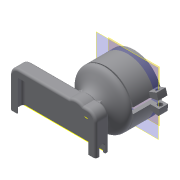
# Autodesk Inventor part: 100_Huawei_Eyepiece_Adapter
Saved by Autodesk Inventor 2019 (Build 230136000, 136)
## iProperties
Created: 2019-05-31
Part Number: 100_Huawei_Eyepiece_Adapter
Material: Generic
Document SubType Name: Modeling
Designer: diederichbenedict
Density: 1 g/cm^3
Appearance: Default
Author: diederichbenedict
Autodesk Inventor part; units mm, degrees
ref_plane "YZ Plane" through (0, 0, 0) normal (1, 0, 0) x (0, 1, 0)
ref_plane "XZ Plane" through (0, 0, 0) normal (0, 1, 0) x (-1, 0, 0)
ref_plane "XY Plane" through (0, 0, 0) normal (0, 0, 1) x (1, 0, 0)
ref_plane "Work Plane1" through (0, 0, -17) normal (0, 0, 1) x (1, 0, 0)
sketch "Sketch1" plane through (0, 0, -17) normal (0, 0, 1) x (1, 0, 0)
  circle A0 centre (0, 0) radius 20.5 construction
  circle A1 centre (0, 0) radius 21
  circle A2 centre (0, 0) radius 24.5
  line L0 (0, 0) -> (4.7167, -24.0417) construction
  line L1 (21, 0) -> (24.5, 0)
  line L2 (24.0417, 4.7167) -> (20.6072, 4.0428)
  point P0 (0, 0)
  point P1 (4.1826, -20.5793)
  point P2 (4.1966, -24.1379)
  point P3 (4.0428, -20.6072)
  dimension "d0" = 42
  dimension "d1" = 49
  constraints: 8 point on circle, 6 end point, 2 centre point, 2 coincident, 1 horizontal, 1 point on line
  measures "d0" diameter of A1
  measures "d1" diameter of A2
extrude "Extrusion1" add sketch "Sketch1" along normal blind 25 contours L1 A2 L2 A1 picked at (23.0923, -1.9696)
sketch "Sketch2" plane through (0, 0, 8) normal (0, 0, 1) x (1, 0, 0)
  arc A0 (20.6072, 4.0428) -> (21, 0) centre (0, 0) ccw projected
  arc A1 (24.0417, 4.7167) -> (24.5, 0) centre (0, 0) ccw projected
  arc A2 (20.6072, 4.0428) -> (21, 0) centre (0, 0) ccw construction
  line L0 (0, 0) -> (-17.3241, 17.3241) construction
  arc A3 (24.0417, 4.7167) -> (24.5, 0) centre (0, 0) ccw construction
  line L1 (0, 0) -> (24.5, 0) construction
  line L2 (-17.3241, 17.3241) -> (0, 0) construction
  line L3 (0, 0) -> (-17.3241, -17.3241) construction
  line L4 (0, 0) -> (24.5, 0) construction
  line L5 (-17.3241, -17.3241) -> (-14.8492, -14.8492)
  line L6 (-17.3241, 17.3241) -> (-14.8492, 14.8492)
  arc A4 (-14.8492, 14.8492) -> (-14.8492, -14.8492) centre (0, 0) ccw
  arc A5 (-17.3241, 17.3241) -> (-17.3241, -17.3241) centre (0, 0) ccw
  line L7 (20.6072, 4.0428) -> (24.0417, 4.7167) projected
  line L8 (24.5, 0) -> (21, 0) projected
  point P0 (0, 0)
  point P1 (0, -21.5)
  point P2 (4.1391, -21.0978)
  point P3 (4.8129, -24.5323)
  point P4 (0, -25)
  dimension "d4" = 135
  dimension "d5" = 225
  constraints: 14 end point, 6 point on circle, 2 centre point, 2 equal length, 2 horizontal, 2 point on line, 1 collinear, 7 other
  measures "d4" angle of L1 L0
extrude "Extrusion2" add sketch "Sketch2" along normal blind 1 contours A0 L5 A1 L6
sketch "Sketch3" plane through (0, 0, 0) normal (1, 0, 0) x (0, 1, 0)
  line L0 (-14.8492, 9) -> (14.8492, 9) projected
  line L1 (14.8492, 9) -> (17.3241, 9) projected
  line L2 (17.3241, 9) -> (-17.3241, 9) projected
  line L3 (-17.3241, 9) -> (-14.8492, 9) projected
  line L4 (24.5, -17) -> (24.5, 8) projected
  line L5 (21, 8) -> (21, -17) projected
  line L6 (-21.0978, -17) -> (-21.0978, 8) projected
  line L7 (-24.5323, -17) -> (-24.5323, 8) projected
  line L8 (2.3, 24.8) -> (2.3, 26.8) projected
  line L9 (-2.1512, 24.8) -> (-2.1512, 31.9)
  line L10 (24.5, 9) -> (17.3241, 9) projected
  line L11 (22.9563, 9) -> (21.506, 13.625) construction
  line L12 (21.506, 13.625) -> (13.0054, 13.9414) construction
  line L13 (13.0054, 13.9414) -> (6.841, 19.4277) construction
  line L14 (6.841, 19.4277) -> (6.841, 24.8) construction
  spline S0 degree 4 poles (22.9563, 9) (21.506, 13.625) (13.0054, 13.9414) (6.841, 19.4277) (6.841, 24.8) knots 1 1 1 1 1 2 2 2 2 2
  line L15 (24.5, 9) -> (24.7161, 14.9037) construction
  line L16 (24.7161, 14.9037) -> (16.0515, 14.6739) construction
  line L17 (16.0515, 14.6739) -> (10.0348, 19.4865) construction
  line L18 (10.0348, 19.4865) -> (10.0348, 24.8) construction
  spline S1 degree 4 poles (24.5, 9) (24.7161, 14.9037) (16.0515, 14.6739) (10.0348, 19.4865) (10.0348, 24.8) knots 1 1 1 1 1 2 2 2 2 2
  line L19 (10.0348, 24.8) -> (6.841, 24.8)
  line L20 (22.9563, 9) -> (24.5, 9)
  line L21 (0, 24.8) -> (0, 0)
  constraints: 8 end point, 2 horizontal, 2 point on line, 2 vertical, 11 other
revolve "Revolution1" add sketch "Sketch3" angle 360 about axis through (0, 0, 24.8) along (0, 0, -1)
sketch "Sketch4" plane through (0, 0, 24.8) normal (0, 0, 1) x (1, 0, 0)
  line L0 (15.2, -132.8) -> (15.2, 2.3) construction
  arc A0 (15.2, 2.3) -> (10.2, 7.3) centre (10.2, 2.3) ccw construction
  line L1 (10.2, 7.3) -> (-50.7, 7.3) construction
  arc A1 (-50.7, 7.3) -> (-55.7, 2.3) centre (-50.7, 2.3) ccw construction
  line L2 (-55.7, 2.3) -> (-55.7, -132.8) construction
  line L3 (16.2, -132.8) -> (16.2, 2.3)
  arc A2 (16.2, 2.3) -> (10.2, 8.3) centre (10.2, 2.3) ccw
  line L4 (10.2, 8.3) -> (-50.7, 8.3)
  arc A3 (-50.7, 8.3) -> (-56.7, 2.3) centre (-50.7, 2.3) ccw
  line L5 (-56.7, 2.3) -> (-56.7, -132.8)
  circle A4 centre (0, 0) radius 10.0348 projected
  circle A5 centre (0, 0) radius 6.841 projected
  line L6 (16.2, -24.5) -> (-56.7, -24.5)
  arc A6 (-17.3241, -17.3241) -> (-17.3241, 17.3241) centre (0, 0) ccw projected
  point P0 (0, 10.0348)
  point P1 (0, 6.841)
  point P2 (5.6397, 8.3)
  point P3 (-5.6397, 8.3)
  dimension "d9" = 1
  constraints: 8 end point, 6 point on circle, 4 point on line, 2 centre point, 1 perpendicular, 1 tangent, 1 vertical alignment, 4 other
  measures "d9" distance between parallel lines of L0 L3
extrude "Extrusion3" add sketch "Sketch4" against normal blind 2
fillet "Fillet1" radius 2 1 edges at (0.003, -10.3555, 22.8)
sketch "Sketch5" plane through (-56.7, -24.5, 24.8) normal (0, -1, 0) x (1, 0, 0)
  line L0 (66.9, 7.1) -> (6, 7.1) construction
  arc A0 (3, 7.1) -> (1, 5.1) centre (3, 5.1) ccw construction
  line L1 (0.5, -2) -> (0.5, -2)
  line L2 (0.5, 2) -> (0.5, 5.8)
  line L3 (0.5, 9.8) -> (0.5, 9.8)
  line L4 (-1.5, 7.8) -> (-1.5, 0)
  line L5 (0.5, 9.8) -> (5.1002, 9.8)
  line L6 (5.1002, 9.8) -> (5.1002, 9.8)
  line L7 (3.1002, 7.8) -> (2.5, 7.8)
  line L8 (0.5, 7.8) -> (0.5, 9.8)
  line L9 (72.9, -2) -> (0, -2) projected
  line L10 (0, 0) -> (72.9, 0) projected
  line L11 (0.5, -2) -> (2.8001, -2)
  line L12 (2.8001, -2) -> (2.8001, 0)
  line L13 (2.8001, 0) -> (2.5, 0)
  line L14 (0.5, 0) -> (0.5, -2)
  arc A1 (0.5, 2) -> (2.5, 0) centre (2.5, 2) ccw
  arc A2 (2.5, 7.8) -> (0.5, 5.8) centre (2.5, 5.8) ccw
  arc A3 (3.1002, 7.8) -> (5.1002, 9.8) centre (3.1002, 9.8) ccw
  arc A4 (0.5, 9.8) -> (-1.5, 7.8) centre (0.5, 7.8) ccw
  arc A5 (-1.5, 0) -> (0.5, -2) centre (0.5, 0) ccw
  point P0 (56.7, -24.8)
  dimension "d14" = 0.7
  dimension "d15" = 0.5
  dimension "d16" = 0
  dimension "d17" = 2
  dimension "d18" = 2
  dimension "d19" = 2
  constraints: 24 end point, 10 point on circle, 10 tangent, 6 parallel, 5 centre point, 5 point on line, 4 equal radius, 3 horizontal, 3 perpendicular
  measures "d14" distance from line of L7 A0.start
  measures "d15" distance from line of L2 A0.end
  measures "d16" distance between parallel lines of L9 L1
  measures "d17" distance between parallel lines of L4 L2
  measures "d18" distance between parallel lines of L7 L5
  measures "d19" radius of A1
sketch "Sketch6" plane through (-56.7, -24.5, 24.8) normal (0, 0, 1) x (1, 0, 0)
  arc A0 (62.3397, 32.8) -> (56.7, 34.5348) centre (56.7, 24.5) ccw projected
  arc A1 (56.7, 34.5348) -> (51.0603, 32.8) centre (56.7, 24.5) ccw projected
  line L0 (51.0603, 32.8) -> (6, 32.8) projected
  arc A2 (6, 32.8) -> (0, 26.8) centre (6, 26.8) ccw projected
  line L1 (0, 26.8) -> (0, 0) projected
  line L2 (0, 0) -> (72.9, 0) projected
  line L3 (72.9, 0) -> (72.9, 26.8) projected
  arc A3 (72.9, 26.8) -> (66.9, 32.8) centre (66.9, 26.8) ccw projected
  line L4 (66.9, 32.8) -> (62.3397, 32.8) projected
  circle A4 centre (56.7, 24.5) radius 6.841 projected
sketch3d "3D Sketch1"
  line L0 (-56.7, -24.5, 24.8) -> (-56.7, 2.3, 24.8)
  arc A0 (-56.7, 2.3, 24.8) -> (-50.7, 8.3, 24.8) centre (-50.7, 2.3, 24.8) ccw
  line L1 (-50.7, 8.3, 24.8) -> (-5.6397, 8.3, 24.8)
  arc A1 (-5.6397, 8.3, 24.8) -> (0, 10.0348, 24.8) centre (0, 0, 24.8) ccw
  arc A2 (0, 10.0348, 24.8) -> (5.6397, 8.3, 24.8) centre (0, 0, 24.8) ccw
  line L2 (5.6397, 8.3, 24.8) -> (10.2, 8.3, 24.8)
  arc A3 (10.2, 8.3, 24.8) -> (16.2, 2.3, 24.8) centre (10.2, 2.3, 24.8) ccw
  line L3 (16.2, 2.3, 24.8) -> (16.2, -24.5, 24.8)
sweep "Sweep1" add profiles "Sketch5" path "3D Sketch1"
sketch "Sketch7" plane through (17.7, -24.5, 32.6) normal (1, 0, 0) x (0, 0, -1)
  line L0 (3.9, -6.0348) -> (3.9, 6.0348) construction
  line L1 (7.8, 0) -> (0, 0) projected
  line L2 (6.4949, -6.0348) -> (6.4949, 6.0348)
  line L3 (1.3051, 6.0348) -> (1.3051, -6.0348)
  arc A0 (1.3051, -6.0348) -> (6.4949, -6.0348) centre (3.9, -6.0348) ccw
  arc A1 (6.4949, 6.0348) -> (1.3051, 6.0348) centre (3.9, 6.0348) ccw
  line L4 (0, 36.0348) -> (7.8, 36.0348) construction
  point P0 (32.6, 24.5)
  point P1 (3.9, 0)
  dimension "d22" = 30
  constraints: 8 end point, 4 point on circle, 4 tangent, 2 centre point, 2 midpoint, 1 parallel, 1 vertical
  measures "d22" distance from line of L4 L0.end
extrude "Extrusion4" cut sketch "Sketch7" against normal blind 4
ref_plane "Work Plane2" through (0, 0, -11) normal (0, 0, -1) x (-1, 0, 0)
sketch "Sketch8" plane through (0, 0, -11) normal (0, 0, -1) x (-1, 0, 0)
  arc A0 (-21, 0) -> (-20.6072, 4.0428) centre (0, 0) ccw projected
  line L0 (-24.5, 0) -> (-21, 0) projected
  arc A1 (-24.5, 0) -> (-24.0417, 4.7167) centre (0, 0) ccw projected
  line L1 (-20.6072, 4.0428) -> (-24.0417, 4.7167) projected
  line L2 (-24.5, 0) -> (-32, 0)
  arc A2 (17.3241, 17.3241) -> (-24.0417, 4.7167) centre (0, 0) ccw projected
  line L3 (-24.0417, 4.7167) -> (-31.4014, 6.1605)
  arc A3 (-32, 0) -> (-31.5138, -5.5567) centre (0, 0) ccw
  arc A4 (0, 22.9563) -> (16.2326, -16.2326) centre (0, 0) ccw projected
  arc A5 (-29.8546, 11.5197) -> (-31.4014, 6.1605) centre (0, 0) ccw
  arc A6 (-24.5, 0) -> (17.3241, -17.3241) centre (0, 0) ccw construction
  line L4 (-31.5138, -5.5567) -> (0, 0) construction
  line L5 (0, 0) -> (-29.8546, 11.5197) construction
  line L6 (-31.5138, -5.5567) -> (-24.1278, -4.2544)
  line L7 (-29.8546, 11.5197) -> (-22.8574, 8.8198)
  line L8 (-20.6072, 4.0428) -> (-24.0417, 4.7167) projected
  arc A7 (-22.8574, 8.8198) -> (-24.0417, 4.7167) centre (0, 0) ccw
  arc A8 (-24.5, 0) -> (-24.1278, -4.2544) centre (0, 0) ccw
  point P0 (0, 0)
  dimension "d27" = 32
  dimension "d28" = 32
  dimension "d29" = 10
  dimension "d30" = 10
  constraints: 12 end point, 11 point on circle, 4 centre point, 2 coincident, 2 concentric, 2 point on line, 1 horizontal
  measures "d27" radius of A3
  measures "d28" radius of A5
  measures "d29" angle of L5 L3
  measures "d30" angle of L2 L4
extrude "Extrusion5" add sketch "Sketch8" along normal mid plane 8 contours A1 L6 A3 L2 | L3 A5 L7 A1
sketch "Sketch9" plane through (29.8546, 11.5197, -7) normal (-0.3599915, 0.9329556, 0) x (0.9329556, 0.3599915, 0)
  line L0 (0, 0) -> (0, 8) projected
  line L1 (-7.5, 8) -> (0, 8) projected
  line L2 (-7.5, 0) -> (-7.5, 8) projected
  line L3 (0, 0) -> (-7.5, 0) projected
  circle A0 centre (-3.5, 4) radius 1.6
  point P0 (-32, -7)
  dimension "d33" = 3.2
  constraints: 1 centre point
  measures "d33" diameter of A0
extrude "Extrusion6" cut sketch "Sketch9" against normal blind 8 contours A0
sketch "Sketch10" plane through (24.1278, -4.2544, -15) normal (-0.1736482, -0.9848078, 0) x (0.9848078, -0.1736482, 0)
  line L0 (5.3546, 8) -> (5.3546, 0) projected
  ellipse E0 centre (2.4994, 4) end of major axis (2.4994, 5.6) minor radius 1.5158 projected
  line L1 (0, 0) -> (0, 8) projected
  line L2 (7.5, 0) -> (0, 0) projected
  line L3 (7.5, 8) -> (7.5, 0) projected
  line L4 (0, 8) -> (7.5, 8) projected
  circle A0 centre (4.0462, 4) radius 2.1
  point P0 (-24.5, 15)
  dimension "d36" = 4.2
  constraints: 1 centre point, 1 other
  measures "d36" diameter of A0
extrude "Extrusion7" cut sketch "Sketch10" against normal blind 8 contours A0 L0 | L0 A0 E0 | E0 A0 picked at (2.645, 4.0388)
body "Solid1"
